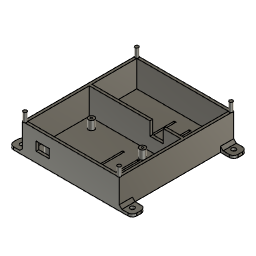
SoftSkillsProjectModel (Autodesk Fusion 360 design; units mm, degrees)
Autodesk Fusion 360 part; units mm, degrees
sketch "Sketch2" plane through (0, 0, 0) normal (0, 0, 1) x (1, 0, 0)
  line L0 (0, 0) -> (110, 0)
  line L1 (110, 0) -> (110, 130)
  line L2 (110, 130) -> (0, 130)
  line L3 (0, 130) -> (0, 0)
  line L4 (3, 127) -> (107, 127)
  line L5 (107, 127) -> (107, 3)
  line L6 (107, 3) -> (3, 3)
  line L7 (3, 3) -> (3, 127)
  line L8 (3, 73) -> (107, 73)
  line L9 (3, 76) -> (107, 76)
  circle A0 centre (16, 62.5) radius 1.4
  circle A1 centre (74, 62.5) radius 1.4
  circle A2 centre (16, 13.5) radius 1.4
  circle A3 centre (74, 13.5) radius 1.4
  circle A4 centre (74, 62.5) radius 3.4
  circle A5 centre (74, 13.5) radius 3.4
  circle A6 centre (16, 13.5) radius 3.4
  circle A7 centre (16, 62.5) radius 3.4
  line L10 (15.6, 3) -> (15.6, 0)
  line L11 (30.6, 3) -> (30.6, 0)
  line L12 (12.5, 66) -> (97.5, 66)
  line L13 (97.5, 66) -> (97.5, 10)
  line L14 (97.5, 10) -> (12.5, 10)
  line L15 (12.5, 10) -> (12.5, 66)
  line L16 (90, 58) -> (92, 58)
  line L17 (92, 58) -> (92, 18)
  line L18 (92, 18) -> (90, 18)
  line L19 (90, 18) -> (90, 58)
  line L20 (73, 58) -> (75, 58)
  line L21 (75, 58) -> (75, 18)
  line L22 (75, 18) -> (73, 18)
  line L23 (73, 18) -> (73, 58)
  line L24 (58, 58) -> (56, 58)
  line L25 (56, 58) -> (56, 18)
  line L26 (56, 18) -> (58, 18)
  line L27 (58, 18) -> (58, 58)
  line L28 (72, 76) -> (72, 73)
  line L29 (87, 76) -> (87, 73)
  dimension "d7" = 110
  dimension "d8" = 130
  dimension "d10" = 3
  dimension "d11" = 3
  dimension "d12" = 3
  dimension "d13" = 3
  dimension "d14" = 70
  dimension "d15" = 3
  dimension "d18" = 2.8
  dimension "d21" = 13
  dimension "d22" = 10.5
  dimension "d23" = 2.8
  dimension "d24" = 10.5
  dimension "d25" = 58
  dimension "d26" = 2.8
  dimension "d27" = 13
  dimension "d28" = 49
  dimension "d29" = 2.8
  dimension "d30" = 49
  dimension "d31" = 58
  dimension "d35" = 6.8
  dimension "d36" = 6.8
  dimension "d37" = 6.8
  dimension "d38" = 6.8
  dimension "d39" = 15
  dimension "d40" = 12.6
  dimension "d41" = 85
  dimension "d42" = 56
  dimension "d43" = 9.5
  dimension "d44" = 7
  dimension "d47" = 2
  dimension "d48" = 40
  dimension "d49" = 15
  dimension "d50" = 15
  dimension "d52" = 2
  dimension "d53" = 2
  dimension "d54" = 15
  dimension "d55" = 15
  dimension "d57" = 15
  dimension "d62" = 20
  constraint horizontal L0
  constraint vertical L1
  constraint horizontal L2
  constraint vertical L3
  constraint coincident L0.start L3.end
  constraint horizontal L4
  constraint vertical L5
  constraint horizontal L6
  constraint vertical L7
  constraint coincident L7 L8.start
  constraint coincident L5 L8.end
  constraint perpendicular L5 L8
  constraint coincident L7 L9.start
  constraint coincident L5 L9.end
  constraint perpendicular L5 L9
  constraint concentric A1 A4
  constraint concentric A3 A5
  constraint concentric A2 A6
  constraint concentric A0 A7
  constraint coincident L6 L10.start
  constraint coincident L0 L10.end
  constraint perpendicular L0 L10
  constraint coincident L6 L11.start
  constraint coincident L0 L11.end
  constraint perpendicular L6 L11
  constraint horizontal L12
  constraint vertical L13
  constraint horizontal L14
  constraint vertical L15
  constraint horizontal L16
  constraint vertical L17
  constraint horizontal L18
  constraint vertical L19
  constraint horizontal L20
  constraint vertical L21
  constraint horizontal L22
  constraint vertical L23
  constraint horizontal L24
  constraint vertical L25
  constraint horizontal L26
  constraint vertical L27
  constraint collinear L16 L20
  constraint collinear L16 L24
  constraint collinear L22 L26
  constraint collinear L18 L26
  constraint coincident L9 L28.start
  constraint coincident L8 L28.end
  constraint perpendicular L9 L28
  constraint coincident L9 L29.start
  constraint coincident L8 L29.end
  constraint perpendicular L8 L29
  measures "d7" distance of L0.start L0.end
  measures "d8" distance of L0.start L2.end
  measures "d10" distance of L1 L5
  measures "d11" distance of L2 L4
  measures "d12" distance of L0 L6
  measures "d13" distance of L3 L7
  measures "d14" distance of L6 L8
  measures "d15" distance of L8 L9
  measures "d18" diameter of A0
  measures "d21" distance of L7 A0.centre
  measures "d22" distance of L8 A0.centre
  measures "d23" diameter of A1
  measures "d24" distance of L8 A1.centre
  measures "d25" distance of A0.centre A1.centre
  measures "d26" diameter of A2
  measures "d27" distance of L7 A2.centre
  measures "d28" distance of A0.centre A2.centre
  measures "d29" diameter of A3
  measures "d30" vertical distance of A1.centre A3.centre
  measures "d31" distance of A2.centre A3.centre
  measures "d35" diameter of A4
  measures "d36" diameter of A5
  measures "d37" diameter of A6
  measures "d38" diameter of A7
  measures "d39" distance of L10 L11
  measures "d40" distance of L7 L10
  measures "d41" distance of L12.start L12.end
  measures "d42" distance of L12.start L14.end
  measures "d43" distance of L7 L15
  measures "d44" distance of L8 L12
  measures "d47" distance of L17.end L18.end
  measures "d48" distance of L16.end L17.end
  measures "d49" distance of L5 L17
  measures "d50" distance of L8 L16
  measures "d52" distance of L25 L27
  measures "d53" distance of L21 L23
  measures "d54" distance of L19 L21
  measures "d55" distance of L23 L27
  measures "d57" distance of L28 L29
  measures "d62" distance of L5 L29
extrude "Extrude2" add sketch "Sketch2" along normal blind 30 contours L0 L1 L2 L3 L4 L5 L6 L7 L10 L11 | L7 L8 L9 L28 | L5 L8 L9 L29 makes body 1
extrude "Extrude1" add sketch "Sketch2" against normal blind 3 separate body contours L0 L1 L2 L3 L4 L5 L6 L7 L10 L11 | L0 L6 L10 L11 | L5 L6 L7 L8 | L7 L8 L9 L28 | L5 L8 L9 L29 | L4 L5 L7 L9 | L8 L9 L28 L29 | A0 | A1 | A2 | A3 | A4 | A5 | A6 | A7 | L12 L13 L14 L15 | L16 L17 L18 L19 | L20 L21 L22 L23 | L24 L25 L26 L27 makes body 2
extrude "Extrude3" cut sketch "Sketch2" against normal blind 3 contours L16 L17 L18 L19 | L20 L21 L22 L23 | L24 L25 L26 L27 bodies 2
extrude "Extrude4" add sketch "Sketch2" along normal blind 15 contours L8 L9 L28 L29 bodies 1 2
extrude "Extrude5" add sketch "Sketch2" along normal blind 10 contours A4 | A5 | A6 | A7 bodies 1
extrude "Extrude6" add sketch "Sketch2" along normal blind 8.5 contours L0 L6 L10 L11 bodies 1
sketch "Sketch3" plane through (30.6, 0, 0) normal (-1, 0, 0) x (0, -1, 0)
  line L0 (-3, 8.5) -> (0, 8.5)
  line L1 (0, 8.5) -> (0, 30)
  line L2 (0, 30) -> (-3, 30)
  line L3 (-3, 30) -> (-3, 8.5)
  line L4 (-3, 18.5) -> (0, 18.5)
  dimension "d80" = 10
  constraint coincident L3 L4.start
  constraint coincident L1 L4.end
  constraint perpendicular L1 L4
  measures "d80" distance of L0 L4
extrude "Extrude7" add sketch "Sketch3" along normal blind 15 contours L1 L2 L3 L4 bodies 1
sketch "Sketch4" plane through (0, 0, 30) normal (0, 0, 1) x (-1, 0, 0)
  line L0 (-107, -3) -> (-3, -3)
  line L1 (-3, -3) -> (-3, -73)
  line L2 (-3, -73) -> (-72, -73)
  line L3 (-72, -73) -> (-72, -76)
  line L4 (-72, -76) -> (-3, -76)
  line L5 (-3, -76) -> (-3, -127)
  line L6 (-3, -127) -> (-107, -127)
  line L7 (-107, -127) -> (-107, -76)
  line L8 (-107, -76) -> (-87, -76)
  line L9 (-87, -76) -> (-87, -73)
  line L10 (-87, -73) -> (-107, -73)
  line L11 (-107, -73) -> (-107, -3)
  line L12 (-110, -130) -> (0, -130)
  line L13 (0, -130) -> (0, 0)
  circle A0 centre (-108.5, -1.5) radius 2
  line L14 (-110, 0) -> (-110, -130)
  line L15 (0, 0) -> (-110, 0)
  circle A1 centre (-1.5, -1.5) radius 2
  circle A2 centre (-108.5, -128.5) radius 2
  line L16 (0, -130) -> (0, 0)
  circle A3 centre (-1.5, -128.5) radius 2
  line L17 (-110, -130) -> (0, -130)
  dimension "d84" = 4
  dimension "d87" = 4
  dimension "d90" = 4
  dimension "d92" = 1.5
  dimension "d93" = 1.5
  dimension "d94" = 1.5
  dimension "d95" = 1.5
  dimension "d96" = 1.5
  dimension "d97" = 1.5
  dimension "d98" = 4
  dimension "d99" = 1.5
  dimension "d100" = 1.5
  measures "d84" diameter of A0
  measures "d87" diameter of A1
  measures "d90" diameter of A2
  measures "d92" distance of L14 A2.centre
  measures "d93" distance of L12 A2.centre
  measures "d94" distance of A0.centre L14
  measures "d95" distance of A0.centre L15
  measures "d96" distance of L15 A1.centre
  measures "d97" distance of A1.centre L16
  measures "d98" diameter of A3
  measures "d99" distance of L16 A3.centre
  measures "d100" distance of A3.centre L17
extrude "Extrude8" add sketch "Sketch4" along normal blind 10 contours L12 L14 A2 L17 | L12 A2 L17 | L14 A2 | L12 L13 L16 A3 L17 | L12 A3 L17 | A0 L14 L15 | A0 L14 | L13 L16 A3 | L13 L15 A1 L16 | L13 A1 L16 | A0 L15 | L15 A1 picked at (-108.9341, -127.7863) picked at (-1.4297, -128.837) picked at (-108.7492, -1.8986) picked at (-1.0117, -1.0691) bodies 1
sketch "Sketch5" plane through (0, 0, 0) normal (0, 0, 1) x (1, 0, 0)
  line L0 (90, 86.5) -> (92, 86.5)
  line L1 (92, 86.5) -> (92, 116.5)
  line L2 (92, 116.5) -> (90, 116.5)
  line L3 (90, 116.5) -> (90, 86.5)
  line L4 (107, 127) -> (107, 3)
  line L5 (3, 127) -> (107, 127)
  line L6 (73, 86.5) -> (75, 86.5)
  line L7 (75, 86.5) -> (75, 116.5)
  line L8 (75, 116.5) -> (73, 116.5)
  line L9 (73, 116.5) -> (73, 86.5)
  line L10 (56, 86.5) -> (58, 86.5)
  line L11 (58, 86.5) -> (58, 116.5)
  line L12 (58, 116.5) -> (56, 116.5)
  line L13 (56, 116.5) -> (56, 86.5)
  line L14 (11, 118) -> (39, 118)
  line L15 (39, 118) -> (39, 92)
  line L16 (39, 92) -> (11, 92)
  line L17 (11, 92) -> (11, 118)
  dimension "d105" = 30
  dimension "d106" = 2
  dimension "d107" = 15
  dimension "d108" = 10.5
  dimension "d109" = 2
  dimension "d110" = 2
  dimension "d111" = 15
  dimension "d112" = 15
  dimension "d117" = 28
  dimension "d118" = 26
  constraint horizontal L0
  constraint vertical L1
  constraint horizontal L2
  constraint vertical L3
  constraint horizontal L6
  constraint vertical L7
  constraint horizontal L8
  constraint vertical L9
  constraint horizontal L10
  constraint vertical L11
  constraint horizontal L12
  constraint vertical L13
  constraint collinear L8 L12
  constraint collinear L2 L12
  constraint collinear L6 L10
  constraint collinear L0 L10
  constraint horizontal L14
  constraint vertical L15
  constraint horizontal L16
  constraint vertical L17
  measures "d105" distance of L0.start L2.end
  measures "d106" distance of L1 L3
  measures "d107" distance of L1 L4
  measures "d108" distance of L2 L5
  measures "d109" distance of L6.start L6.end
  measures "d110" distance of L10.start L10.end
  measures "d111" distance of L3 L7
  measures "d112" distance of L9 L11
  measures "d117" distance of L14.start L14.end
  measures "d118" distance of L14.start L16.end
extrude "Extrude9" cut sketch "Sketch5" against normal blind 3 contours L0 L1 L2 L3 | L6 L7 L8 L9 | L10 L11 L12 L13 bodies 1
sketch "Sketch7" plane through (0, 0, 0) normal (0, 0, 1) x (1, 0, 0)
  line L0 (-161.2037, 91.5) -> (-31.2037, 91.5)
  line L1 (-31.2037, 91.5) -> (-31.2037, -58.5)
  line L2 (-31.2037, -58.5) -> (-161.2037, -58.5)
  line L3 (-161.2037, -58.5) -> (-161.2037, 91.5)
  line L4 (-161.2037, -58.5) -> (-31.2037, 91.5) construction
  line L5 (-31.2037, -58.5) -> (-161.2037, 91.5) construction
  circle A0 centre (-149.7037, -47) radius 2.5
  circle A1 centre (-42.7037, -47) radius 2.5
  circle A2 centre (-42.7037, 80) radius 2.5
  circle A3 centre (-149.7037, 80) radius 2.5
  line L6 (-145.2037, -42.5) -> (-145.2037, 75.5)
  line L7 (-145.2037, 75.5) -> (-47.2037, 75.5)
  line L8 (-47.2037, 75.5) -> (-47.2037, -42.5)
  line L9 (-47.2037, -42.5) -> (-145.2037, -42.5)
  dimension "d120" = 130
  dimension "d121" = 150
  dimension "d125" = 5
  dimension "d126" = 11.5
  dimension "d127" = 11.5
  dimension "d128" = 5
  dimension "d129" = 11.5
  dimension "d130" = 11.5
  dimension "d131" = 5
  dimension "d132" = 5
  dimension "d133" = 11.5
  dimension "d134" = 11.5
  dimension "d135" = 11.5
  dimension "d136" = 11.5
  dimension "d217" = 16
  dimension "d236" = 118
  dimension "d237" = 98
  constraint horizontal L0
  constraint vertical L1
  constraint horizontal L2
  constraint vertical L3
  measures "d120" distance of L1.end L2.end
  measures "d121" distance of L0.start L2.end
  measures "d125" diameter of A0
  measures "d126" distance of L2 A0.centre
  measures "d127" distance of L3 A0.centre
  measures "d128" diameter of A1
  measures "d129" distance of L1 A1.centre
  measures "d130" distance of L2 A1.centre
  measures "d131" diameter of A2
  measures "d132" diameter of A3
  measures "d133" distance of L0 A3.centre
  measures "d134" distance of L3 A3.centre
  measures "d135" distance of L1 A2.centre
  measures "d136" distance of L0 A2.centre
  measures "d236" distance of L6.start L6.end
  measures "d237" distance of L6.start L8.end
extrude "Extrude10" add sketch "Sketch7" along normal blind 10 separate body contours L0 L1 L2 L3 | A0 | A1 | A2 | A3 | L6 L7 L8 L9 makes body 3
chamfer "Chamfer1" distance 10 angle 45 4 edges at (-161.2037, 16.5, 10) (-96.2037, -58.5, 10) (-31.2037, 16.5, 10) (-96.2037, 91.5, 10) on bodies 3
extrude "Extrude11" cut sketch "Sketch7" along normal blind 5 contours A0 | A1 | A2 | A3 bodies 3
sketch "Sketch9" plane through (0, 0, -3) normal (0, 0, -1) x (1, 0, 0)
  line L0 (56, -86.5) -> (58, -86.5)
  line L1 (58, -86.5) -> (58, -116.5)
  line L2 (58, -116.5) -> (56, -116.5)
  line L3 (56, -116.5) -> (56, -86.5)
  line L4 (73, -86.5) -> (75, -86.5)
  line L5 (75, -86.5) -> (75, -116.5)
  line L6 (75, -116.5) -> (73, -116.5)
  line L7 (73, -116.5) -> (73, -86.5)
  line L8 (90, -86.5) -> (92, -86.5)
  line L9 (92, -86.5) -> (92, -116.5)
  line L10 (92, -116.5) -> (90, -116.5)
  line L11 (90, -116.5) -> (90, -86.5)
  line L12 (75, -18) -> (75, -58)
  line L13 (75, -58) -> (73, -58)
  line L14 (73, -58) -> (73, -18)
  line L15 (73, -18) -> (75, -18)
  line L16 (58, -58) -> (56, -58)
  line L17 (56, -58) -> (56, -18)
  line L18 (56, -18) -> (58, -18)
  line L19 (58, -18) -> (58, -58)
  line L20 (92, -18) -> (92, -58)
  line L21 (92, -58) -> (90, -58)
  line L22 (90, -58) -> (90, -18)
  line L23 (90, -18) -> (92, -18)
  line L24 (0, 0) -> (0, -130)
  line L25 (0, -130) -> (110, -130)
  line L26 (110, -130) -> (110, 0)
  line L27 (110, 0) -> (0, 0)
  line L28 (110, 0) -> (120, 0)
  line L29 (125, -5) -> (125, -10)
  line L30 (120, -15) -> (110, -15)
  line L31 (110, -15) -> (110, 0)
  circle A0 centre (117.5, -7.5) radius 2.5
  arc A1 (125, -5) -> (120, 0) centre (120, -5) ccw
  circle A2 centre (117.5, -7.5) radius 2.5
  arc A3 (120, -15) -> (125, -10) centre (120, -10) ccw
  circle A4 centre (117.5, -122.5) radius 2.5
  arc A5 (125, -120) -> (120, -115) centre (120, -120) ccw
  line L32 (120, -130) -> (110, -130)
  line L33 (110, -130) -> (110, -115)
  arc A6 (120, -130) -> (125, -125) centre (120, -125) ccw
  line L34 (125, -120) -> (125, -125)
  line L35 (110, -115) -> (120, -115)
  line L36 (-10, -115) -> (0, -115)
  line L37 (-15, -125) -> (-15, -120)
  circle A7 centre (-7.5, -122.5) radius 2.5
  arc A8 (-10, -115) -> (-15, -120) centre (-10, -120) ccw
  line L38 (0, -115) -> (0, -130)
  arc A9 (-15, -125) -> (-10, -130) centre (-10, -125) ccw
  line L39 (0, -130) -> (-10, -130)
  circle A10 centre (-7.5, -7.5) radius 2.5
  arc A11 (-10, 0) -> (-15, -5) centre (-10, -5) ccw
  line L40 (-10, 0) -> (0, 0)
  line L41 (-15, -10) -> (-15, -5)
  arc A12 (-15, -10) -> (-10, -15) centre (-10, -10) ccw
  line L42 (0, 0) -> (0, -15)
  line L43 (0, -15) -> (-10, -15)
  point P0 (125, 0)
  point P1 (125, 0)
  point P2 (110, -115)
  point P3 (0, -130)
  point P4 (-15, -130)
  point P5 (-19.7326, -130.5247)
  point P6 (0, -15)
  point P7 (-15, -15)
  point P8 (-20.5125, -15.7908)
  dimension "d144" = 10
  dimension "d145" = 10
  dimension "d153" = 5
  dimension "d154" = 5
  dimension "d155" = 5
  dimension "d158" = 5
  dimension "d159" = 5
  dimension "d161" = 5
  dimension "d164" = 10
  dimension "d165" = 5
  dimension "d166" = 5
  dimension "d167" = 5
  dimension "d168" = 5
  dimension "d169" = 5
  dimension "d174" = 10
  dimension "d175" = 10
  dimension "d176" = 5
  dimension "d177" = 5
  dimension "d178" = 5
  dimension "d185" = 10
  dimension "d186" = 10
  dimension "d187" = 5
  dimension "d188" = 5
  dimension "d189" = 5
  constraint horizontal L28
  constraint vertical L29
  constraint horizontal L30
  constraint vertical L31
  constraint coincident L26.end L27.start
  constraint coincident P1 L29
  constraint coincident P1 L28
  constraint tangent L29 A1
  constraint tangent L28 A1
  constraint horizontal L35
  constraint vertical L34
  constraint horizontal L32
  constraint vertical L33
  constraint coincident P2 L33.end
  constraint tangent L32 A6
  constraint tangent A6 L34
  constraint tangent A5 L34
  constraint tangent A5 L35
  constraint collinear L31 L33
  constraint coincident L25.end L32
  constraint coincident P3 L24.end
  constraint tangent L36 A8
  constraint tangent L37 A8
  constraint coincident P4 L37
  constraint coincident P4 L39
  constraint tangent L37 A9
  constraint tangent A9 L39
  constraint collinear L25 L39
  constraint collinear L24 L38
  constraint coincident P6 L42.end
  constraint coincident P7 L41
  constraint coincident P7 L43
  constraint tangent L41 A12
  constraint tangent A12 L43
  constraint coincident L24.start L27.end
  constraint coincident A11.start L40.start
  measures "d153" diameter of A0
  measures "d158" radius of A1
  measures "d159" diameter of A2
  measures "d161" radius of A3
  measures "d165" diameter of A4
  measures "d168" radius of A6
  measures "d169" radius of A5
  measures "d176" diameter of A7
  measures "d187" diameter of A10
extrude "Extrude12" add sketch "Sketch9" against normal blind 3 contours L24 A11 L40 L41 A12 L42 L43 | L26 L28 L29 L30 L31 A1 A3 | L24 L36 L37 A8 L38 A9 L39 | L26 A5 L32 L33 A6 L34 L35 bodies 1
chamfer "Chamfer2" distance 3 angle 45 4 edges at (0, 7.5, 0) (0, 122.5, 0) (110, 7.5, 0) (110, 122.5, 0) on bodies 1
extrude "Extrude13" add 1 faces at (74.3421, 62.9565, 0) along direction (0, 0, 1) blind 10 on bodies 1 bodies 1
hole "Hole1" at (74, 62.5, 10) direction (0, 0, -1) diameter 2.175 depth 10 tip angle 118 bodies 1
thread "Thread1" "ISO Metric profile 2.6 M2.6x0.45 6H"
extrude "Extrude14" add sketch "Sketch2" along normal blind 10 contours A0 bodies 1
hole "Hole2" at (16, 62.5, 10) direction (0, 0, -1) diameter 2.175 depth 10 tip angle 118 bodies 1
thread "Thread2" "ISO Metric profile 2.6 M2.6x0.45 6H"
extrude "Extrude15" add sketch "Sketch2" along normal blind 10 contours A2 bodies 1
hole "Hole3" at (16, 13.5, 10) direction (0, 0, -1) diameter 2.175 depth 10 tip angle 118 bodies 1
thread "Thread3" "ISO Metric profile 2.6 M2.6x0.45 6H"
extrude "Extrude16" add sketch "Sketch2" along normal blind 10 contours A3 bodies 1
hole "Hole4" at (74, 13.5, 10) direction (0, 0, -1) diameter 2.175 depth 10 tip angle 118 bodies 1
thread "Thread4" "ISO Metric profile 2.6 M2.6x0.45 6H"
sketch "Sketch10" plane through (0, 0, 0) normal (1, 0, 0) x (0, 1, 0)
extrude "Extrude17" cut sketch "Sketch7" along normal blind 5 contours L6 L7 L8 L9 bodies 3
sketch "Sketch11" plane through (0, 0, 0) normal (0, 0, 1) x (1, 0, 0)
  line L0 (-305, 90) -> (-175, 90)
  line L1 (-175, 90) -> (-175, -60)
  line L2 (-175, -60) -> (-305, -60)
  line L3 (-305, -60) -> (-305, 90)
  circle A0 centre (-293.5, -48.5) radius 2.75
  circle A1 centre (-186.5, -48.5) radius 2.75
  circle A2 centre (-293.5, 78.5) radius 2.75
  circle A3 centre (-186.5, 78.5) radius 2.75
  point P0 (-293.5, -48.5)
  dimension "d220" = 130
  dimension "d221" = 150
  dimension "d222" = 11.5
  dimension "d223" = 11.5
  dimension "d224" = 5.5
  dimension "d225" = 5.5
  dimension "d226" = 11.5
  dimension "d227" = 11.5
  dimension "d228" = 5.5
  dimension "d229" = 11.5
  dimension "d230" = 11.5
  dimension "d231" = 5.5
  dimension "d232" = 11.5
  dimension "d233" = 11.5
  constraint horizontal L0
  constraint vertical L1
  constraint horizontal L2
  constraint vertical L3
  measures "d220" distance of L0.start L0.end
  measures "d221" distance of L0.start L2.end
  measures "d222" distance of L2 P0
  measures "d223" distance of L3 P0
  measures "d224" diameter of A0
  measures "d225" diameter of A1
  measures "d226" distance of L2 A1.centre
  measures "d227" distance of L1 A1.centre
  measures "d228" diameter of A2
  measures "d229" distance of L3 A2.centre
  measures "d230" distance of L0 A2.centre
  measures "d231" diameter of A3
  measures "d232" distance of L0 A3.centre
  measures "d233" distance of L1 A3.centre
sketch "Sketch12" plane through (0, 0, 0) normal (0, 0, 1) x (1, 0, 0)
sketch "Sketch13" plane through (0, 0, 0) normal (0, 0, 1) x (1, 0, 0)
  line L0 (-234.4601, -236.7552) -> (-104.4601, -236.7552)
  line L1 (-104.4601, -236.7552) -> (-104.4601, -86.7552)
  line L2 (-104.4601, -86.7552) -> (-234.4601, -86.7552)
  line L3 (-234.4601, -86.7552) -> (-234.4601, -236.7552)
  dimension "d234" = 130
  dimension "d235" = 150
  constraint horizontal L0
  constraint vertical L1
  constraint horizontal L2
  constraint vertical L3
  measures "d234" distance of L0.start L0.end
  measures "d235" distance of L0.start L2.end
copy_body "Body->Comp1" bodies 1 removing the originals makes body 4 in component "Component"
component "Component" placed x (1, 0, 0) y (0, 1, 0) z (0, 0, 1) at (0, 0, 0)
hidden bodies 3
equation "WallThickness = 3 mm"
equation "HoleDiameter = 2.8 mm"
equation "PiHoleDistanceLength = 58 mm"
equation "PiHoleDistanceWidth = 49 mm"
equation "BoxLength = 110 mm"
equation "BoxWidth = 130 mm"
equation "d7 = BoxLength"
equation "d8 = BoxWidth"
equation "PiCompartmentWidth = 70 mm"
equation "d10 = WallThickness"
equation "d11 = WallThickness"
equation "d12 = WallThickness"
equation "d13 = WallThickness"
equation "d14 = PiCompartmentWidth"
equation "d15 = WallThickness"
equation "PiWidth = 56 mm"
equation "PiLength = 85 mm"
equation "d18 = HoleDiameter"
equation "PiHoleToLongSide = 3.5 mm"
equation "PiHoleToShortSide = 3.5 mm"
equation "d21 = ( BoxLength - 2 * WallThickness - PiLength ) / 2 + PiHoleToShortSide"
equation "d22 = ( PiCompartmentWidth - PiWidth ) / 2 + PiHoleToLongSide"
equation "d23 = HoleDiameter"
equation "d24 = d22"
equation "d25 = PiHoleDistanceLength"
equation "d26 = HoleDiameter"
equation "d27 = d21"
equation "d28 = PiHoleDistanceWidth"
equation "d29 = HoleDiameter"
equation "d30 = d28"
equation "d31 = d25"
equation "PiPowerOffset = 10.6 mm"
equation "PiPowerWidth = 15 mm"
equation "HoleCylinderWidth = 2 mm"
equation "d35 = HoleDiameter + HoleCylinderWidth * 2"
equation "d36 = d35"
equation "d37 = d35"
equation "d38 = d37"
equation "d39 = PiPowerWidth"
equation "d40 = ( BoxLength - 2 * WallThickness - PiLength ) / 2 + ( PiPowerOffset - PiPowerWidth / 2 )"
equation "d41 = PiLength"
equation "d42 = PiWidth"
equation "d43 = ( BoxLength - 2 * WallThickness - PiLength ) / 2"
equation "d44 = ( PiCompartmentWidth - PiWidth ) / 2"
equation "AirVentWidth = 2 mm"
equation "AirWentLength = 40 mm"
equation "d47 = AirVentWidth"
equation "d48 = AirWentLength"
equation "d49 = AirVentDistance"
equation "d50 = ( PiCompartmentWidth - AirWentLength ) / 2"
equation "d52 = d47"
equation "d53 = d47"
equation "d54 = d49"
equation "d55 = d49"
equation "WireHoleWidth = 15 mm"
equation "d57 = WireHoleWidth"
equation "AirVentDistance = 15 mm"
equation "WireHoleOffset = 20 mm"
equation "d62 = WireHoleOffset"
equation "FloorThickness = 3 mm"
equation "d64 = -FloorThickness"
equation "WallHeight = 30 mm"
equation "ScrewHeight = 10 mm"
equation "d68 = WallHeight"
equation "d70 = -FloorThickness"
equation "WireHoleHeight = 15 mm"
equation "d73 = WallHeight - WireHoleHeight"
equation "d75 = ScrewHeight"
equation "PiPowerHeight = 10 mm"
equation "d78 = ScrewHeight - ( 0.15 * PiPowerHeight )"
equation "d80 = PiPowerHeight"
equation "d81 = PiPowerWidth"
equation "RoofPinDiameter = 4 mm"
equation "d84 = RoofPinDiameter"
equation "d85 = WallThickness / 2"
equation "d86 = WallThickness / 2"
equation "d87 = d84"
equation "d90 = d84"
equation "d92 = WallThickness / 2"
equation "d93 = d92"
equation "d94 = d92"
equation "d95 = d92"
equation "d96 = d92"
equation "d97 = d92"
equation "d98 = d84"
equation "d99 = d92"
equation "d100 = d92"
equation "RoofPinHeight = 10 mm"
equation "d102 = RoofPinHeight"
equation "SensorAirVentLength = 30 mm"
equation "d105 = SensorAirVentLength"
equation "d106 = AirVentWidth"
equation "d107 = AirVentDistance"
equation "d108 = ( BoxWidth - PiCompartmentWidth - 3 * WallThickness - SensorAirVentLength ) / 2"
equation "d109 = AirVentWidth"
equation "d110 = AirVentWidth"
equation "d111 = d107"
equation "d112 = d107"
equation "d113 = -FloorThickness"
equation "SensorWidth = 26 mm"
equation "SensorLength = 28 mm"
equation "d117 = SensorLength"
equation "d118 = SensorWidth"
equation "RoofOverhang = 10 mm"
equation "d120 = BoxLength + 2 * RoofOverhang"
equation "d121 = BoxWidth + 2 * RoofOverhang"
equation "d122 = RoofHeight"
equation "d124 = RoofBevel"
equation "d125 = RoofPinDiameter + 1 mm"
equation "d126 = RoofOverhang + WallThickness / 2"
equation "d127 = d126"
equation "d128 = d125"
equation "d129 = d127"
equation "d130 = d127"
equation "d131 = d125"
equation "d132 = d125"
equation "d133 = d126"
equation "d134 = d126"
equation "d135 = d126"
equation "d136 = d126"
equation "RoofPinInsetDepth = 5 mm"
equation "d138 = RoofPinInsetDepth"
equation "RoofHeight = 10 mm"
equation "RoofBevel = 10 mm"
equation "BoxStandPinDiameter = 5 mm"
equation "FootRectSize = 10 mm"
equation "d144 = FootRectSize"
equation "d145 = FootRectSize"
equation "FootScrewHole = 5 mm"
equation "d153 = FootScrewHole"
equation "d154 = FootRectSize / 2"
equation "d155 = FootRectSize / 2"
equation "FootCornerCircleDiameter = 5 mm"
equation "d158 = FootCornerCircleDiameter"
equation "d159 = FootScrewHole"
equation "d161 = FootCornerCircleDiameter"
equation "d164 = FootRectSize"
equation "d165 = FootScrewHole"
equation "d166 = FootRectSize / 2"
equation "d167 = FootRectSize / 2"
equation "d168 = FootCornerCircleDiameter"
equation "d169 = FootCornerCircleDiameter"
equation "d174 = FootRectSize"
equation "d175 = FootRectSize"
equation "d176 = FootScrewHole"
equation "d177 = FootRectSize / 2"
equation "d178 = FootRectSize / 2"
equation "d185 = FootRectSize"
equation "d186 = FootRectSize"
equation "d187 = FootScrewHole"
equation "d188 = FootRectSize / 2"
equation "d189 = FootRectSize / 2"
equation "d193 = -FloorThickness"
equation "FootBevel = 3 mm"
equation "d196 = FootBevel"
equation "d197 = ScrewHeight"
equation "d199 = ScrewHeight"
equation "d202 = ScrewHeight"
equation "d204 = ScrewHeight"
equation "d207 = ScrewHeight"
equation "d209 = ScrewHeight"
equation "d212 = ScrewHeight"
equation "d214 = ScrewHeight"
equation "d217 = RoofOverhang + WallThickness * 2"
equation "d218 = RoofPinInsetDepth"
equation "d220 = BoxLength + 2 * RoofOverhang"
equation "d221 = BoxWidth + RoofOverhang * 2"
equation "d222 = RoofOverhang + WallThickness / 2"
equation "d223 = RoofOverhang + WallThickness / 2"
equation "d224 = RoofPinDiameter + 1.5 mm"
equation "d225 = RoofPinDiameter + 1.5 mm"
equation "d226 = RoofOverhang + WallThickness / 2"
equation "d227 = RoofOverhang + WallThickness / 2"
equation "d228 = RoofPinDiameter + 1.5 mm"
equation "d229 = RoofOverhang + WallThickness / 2"
equation "d230 = RoofOverhang + WallThickness / 2"
equation "d231 = RoofPinDiameter + 1.5 mm"
equation "d232 = RoofOverhang + WallThickness / 2"
equation "d233 = RoofOverhang + WallThickness / 2"
equation "d234 = BoxLength + 2 * RoofOverhang"
equation "d235 = BoxWidth + RoofOverhang * 2"
